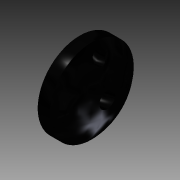
# Autodesk Inventor part: Flexiwheel Hub - Out Side
Saved by Autodesk Inventor 2014 (Build 180170000, 170)
## iProperties
Created: 2014-02-03
Part Number: Flexiwheel Hub - Out Side
Material: Generic
Document SubType Name: Modeling
Designer: Spooner
Density: 1 g/cm^3
Appearance: Black
Author: Spooner
Autodesk Inventor part; units mm, degrees
ref_plane "XZ Plane" through (0, 0, 0) normal (0, 1, 0) x (-1, 0, 0)
sketch "Sketch1" plane through (0, 0, 0) normal (0, 0, 1) x (1, 0, 0)
  line L0 (0, 0) -> (-8.052, 0) construction
  line L1 (-6.096, 2.032) -> (5.08, 2.032)
  line L2 (-6.096, 2.032) -> (-6.096, 3.2258)
  line L3 (-6.096, 3.2258) -> (0, 3.2258)
  line L4 (0, 3.2258) -> (0, 6.9342)
  line L5 (0, 6.9342) -> (-3.81, 6.9342)
  line L6 (-3.81, 6.9342) -> (-3.81, 13.5128)
  line L7 (-3.81, 13.5128) -> (0, 13.5128)
  arc A0 (5.08, 2.032) -> (0, 13.5128) centre (-15.0256, 0) ccw
  dimension "d0" = 2.032
  dimension "d1" = 13.5128
  dimension "d2" = 6.096
  dimension "d3" = 3.2258
  dimension "d4" = 3.81
  dimension "d5" = 6.9342
  dimension "d7" = 5.08
  constraints: 16 end point, 5 parallel, 2 perpendicular, 2 point on circle, 2 vertical alignment, 1 centre point, 1 horizontal, 1 point on line
  measures "d0" distance between parallel lines of L0 L1
  measures "d1" distance between parallel lines of L0 L7
  measures "d2" distance from line of L2 L7.end
  measures "d3" distance between parallel lines of L0 L3
  measures "d4" distance from line of L7.end L6
  measures "d5" distance between parallel lines of L0 L5
  measures "d7" horizontal distance of L0.start L1.end
revolve "Revolution1" add sketch "Sketch1" angle 360 about axis through (0, 0, 0) along (-1, 0, 0)
ref_plane "Work Plane3" through (3.9124, 0, 0) normal (1, 0, 0) x (0, 1, 0)
ref_plane "Work Plane2" through (5.1824, 0, 0) normal (1, 0, 0) x (0, 1, 0)
sketch "Sketch4" plane through (-3.81, 0, 0) normal (-1, 0, 0) x (0, 0, 1)
  circle A0 centre (0, 10.16) radius 1.7272 projected
extrude "Extrusion3" cut sketch "Sketch4" against normal through all
sketch "Sketch5" plane through (-6.096, 0, 0) normal (-1, 0, 0) x (0, 0, 1)
  circle A0 centre (0, 0) radius 2.032 projected
  circle A1 centre (0, 0) radius 3.2258 projected
  circle A2 centre (0, 0) radius 1.143
  dimension "d18" = 2.286
  constraints: 1 centre point, 1 coincident
  measures "d18" diameter of A2
extrude "Extrusion4" add sketch "Sketch5" against normal up to surface contours A0
ref_plane "Work Plane4" through (-2.921, 0, 0) normal (-1, 0, 0) x (0, 0, 1)
sketch "Sketch6" plane through (-2.921, 0, 0) normal (-1, 0, 0) x (0, 0, 1)
  circle A0 centre (0, 0) radius 2.54
  dimension "d22" = 5.08
  constraints: 1 centre point, 1 coincident
  measures "d22" diameter of A0
extrude "Extrusion5" cut sketch "Sketch6" against normal through all
chamfer "Chamfer1" distance 1.27 angle 45 1 edges at (-2.921, 0, -1.143)
body "Solid1"
